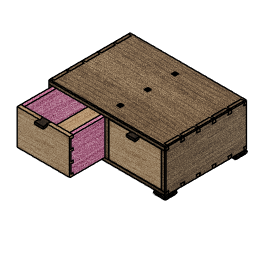
Drawer Box 2019 (Autodesk Fusion 360 design; units mm, degrees)
Autodesk Fusion 360 part; units mm, degrees
note: some values were not read from the file. Chosen so that the rebuilt part matches the saved one: which face or edge a step refers to. Set by a fixed rule: which sketch regions a step uses.
(part 1 of 2)
sketch "Sketch1" plane through (0, 0, 0) normal (0, 1, 0) x (1, 0, 0) in component "Bottom"
  line L0 (0, 0) -> (254, 0)
  line L1 (254, 0) -> (254, -177.8)
  line L2 (254, -177.8) -> (0, -177.8)
  line L3 (0, -177.8) -> (0, 0)
  dimension "d8" = 254
  dimension "d9" = 177.8
  constraint horizontal L0
  constraint vertical L1
  constraint horizontal L2
  constraint vertical L3
  constraint coincident L0.start L3.end
  measures "d8" distance of L1.end L2.end
  measures "d9" distance of L0.start L2.end
extrude "Extrude1" add sketch "Sketch1" along normal blind 15.875 makes body 1 in component "Bottom"
ref_plane "WorkPlane1" through (127, 7.9375, 88.9) normal (1, 0, 0) x (0, 0, -1) in component "Bottom"
ref_plane "WorkPlane3" through (127, 7.9375, 88.9) normal (0, 0, 1) x (1, 0, 0) in component "Bottom"
sketch "Sketch2" plane through (0, 0, 0) normal (-1, 0, 0) x (0, 0, 1) in component "Bottom"
  line L0 (0, 0) -> (177.8, 0)
  line L1 (177.8, 0) -> (177.8, 15.875)
  line L2 (177.8, 15.875) -> (0, 15.875)
  line L3 (0, 15.875) -> (0, 0)
  line L4 (76.2, 15.875) -> (73.6209, 7.9375)
  line L5 (73.6209, 7.9375) -> (104.1791, 7.9375)
  line L6 (104.1791, 7.9375) -> (101.6, 15.875)
  line L7 (144.4625, 15.875) -> (141.8834, 7.9375)
  line L8 (141.8834, 7.9375) -> (172.4416, 7.9375)
  line L9 (172.4416, 7.9375) -> (169.8625, 15.875)
  line L10 (110.3313, 15.875) -> (107.7522, 7.9375)
  line L11 (107.7522, 7.9375) -> (138.3103, 7.9375)
  line L12 (138.3103, 7.9375) -> (135.7312, 15.875)
  line L13 (42.0688, 15.875) -> (39.4897, 7.9375)
  line L14 (39.4897, 7.9375) -> (70.0478, 7.9375)
  line L15 (70.0478, 7.9375) -> (67.4688, 15.875)
  line L16 (7.9375, 15.875) -> (5.3584, 7.9375)
  line L17 (5.3584, 7.9375) -> (35.9166, 7.9375)
  line L18 (35.9166, 7.9375) -> (33.3375, 15.875)
  line L19 (76.2, 15.875) -> (101.6, 15.875)
  line L20 (144.4625, 15.875) -> (169.8625, 15.875)
  line L21 (110.3313, 15.875) -> (135.7312, 15.875)
  line L22 (42.0688, 15.875) -> (67.4688, 15.875)
  line L23 (7.9375, 15.875) -> (33.3375, 15.875)
  dimension "d12" = 72
  dimension "d13" = 72
  dimension "d17" = 68.2625
  dimension "d18" = 0
  dimension "d22" = 25.4
  dimension "d23" = 7.9375
  constraint coincident L2 L4.start
  constraint parallel L2 L5
  constraint coincident L2 L6.end
  constraint parallel L2 L19
  constraint midpoint L2 L19
  measures "d12" angle of L4 L5
  measures "d13" angle of L5 L6
  measures "d22" distance of L4.start L6.end
  measures "d23" distance of L5 L19
extrude "Extrude2" cut sketch "Sketch2" against normal blind 7.9375 contours L2 L16 L17 L18 L23 | L2 L7 L8 L9 L20 | L2 L13 L14 L15 L22 | L2 L10 L11 L12 L21 | L2 L4 L5 L6 L19 bodies 1 in component "Bottom"
mirror "Mirror1" about plane through (127, 7.9375, 88.9) normal (1, 0, 0) of "Extrude2" in component "Bottom"
sketch "Sketch3" plane through (0, 15.875, 0) normal (0, 1, 0) x (-1, 0, 0) in component "Bottom"
  line L0 (-246.0625, 76.2) -> (-254, 76.2)
  line L1 (-254, 76.2) -> (-254, 67.4688)
  line L2 (-254, 67.4688) -> (-246.0625, 67.4688)
  line L3 (-246.0625, 67.4688) -> (-246.0625, 42.0688)
  line L4 (-246.0625, 42.0688) -> (-254, 42.0688)
  line L5 (-254, 42.0688) -> (-254, 33.3375)
  line L6 (-254, 33.3375) -> (-246.0625, 33.3375)
  line L7 (-246.0625, 33.3375) -> (-246.0625, 7.9375)
  line L8 (-246.0625, 7.9375) -> (-254, 7.9375)
  line L9 (-254, 7.9375) -> (-254, 0)
  line L10 (-254, 0) -> (0, 0)
  line L11 (0, 0) -> (0, 7.9375)
  line L12 (0, 7.9375) -> (-7.9375, 7.9375)
  line L13 (-7.9375, 7.9375) -> (-7.9375, 33.3375)
  line L14 (-7.9375, 33.3375) -> (0, 33.3375)
  line L15 (0, 33.3375) -> (0, 42.0688)
  line L16 (0, 42.0688) -> (-7.9375, 42.0688)
  line L17 (-7.9375, 42.0688) -> (-7.9375, 67.4688)
  line L18 (-7.9375, 67.4688) -> (0, 67.4688)
  line L19 (0, 67.4688) -> (0, 76.2)
  line L20 (0, 76.2) -> (-7.9375, 76.2)
  line L21 (-7.9375, 76.2) -> (-7.9375, 101.6)
  line L22 (-7.9375, 101.6) -> (0, 101.6)
  line L23 (0, 101.6) -> (0, 110.3313)
  line L24 (0, 110.3313) -> (-7.9375, 110.3313)
  line L25 (-7.9375, 110.3313) -> (-7.9375, 135.7312)
  line L26 (-7.9375, 135.7313) -> (0, 135.7313)
  line L27 (0, 135.7313) -> (0, 144.4625)
  line L28 (0, 144.4625) -> (-7.9375, 144.4625)
  line L29 (-7.9375, 144.4625) -> (-7.9375, 169.8625)
  line L30 (-7.9375, 169.8625) -> (0, 169.8625)
  line L31 (0, 169.8625) -> (0, 177.8)
  line L32 (0, 177.8) -> (-254, 177.8)
  line L33 (-254, 177.8) -> (-254, 169.8625)
  line L34 (-254, 169.8625) -> (-246.0625, 169.8625)
  line L35 (-246.0625, 169.8625) -> (-246.0625, 144.4625)
  line L36 (-246.0625, 144.4625) -> (-254, 144.4625)
  line L37 (-254, 144.4625) -> (-254, 135.7313)
  line L38 (-254, 135.7313) -> (-246.0625, 135.7313)
  line L39 (-246.0625, 135.7313) -> (-246.0625, 110.3313)
  line L40 (-246.0625, 110.3313) -> (-254, 110.3313)
  line L41 (-254, 110.3313) -> (-254, 101.6)
  line L42 (-254, 101.6) -> (-246.0625, 101.6)
  line L43 (-246.0625, 101.6) -> (-246.0625, 76.2)
  line L44 (-127, 0) -> (-127, 177.8) construction
  line L45 (-123.0312, 84.9313) -> (-130.9688, 84.9313)
  line L46 (-130.9688, 84.9313) -> (-130.9688, 92.8688)
  line L47 (-130.9688, 92.8688) -> (-123.0312, 92.8688)
  line L48 (-123.0312, 92.8688) -> (-123.0312, 84.9313)
  line L49 (-130.9688, 84.9313) -> (-123.0312, 92.8688) construction
  line L50 (-123.0312, 25.6646) -> (-130.9688, 25.6646)
  line L51 (-123.0312, 33.6021) -> (-123.0312, 25.6646)
  line L52 (-130.9688, 33.6021) -> (-123.0312, 33.6021)
  line L53 (-130.9688, 25.6646) -> (-130.9688, 33.6021)
  line L54 (-123.0312, 144.1979) -> (-130.9688, 144.1979)
  line L55 (-123.0312, 152.1354) -> (-123.0312, 144.1979)
  line L56 (-130.9688, 152.1354) -> (-123.0312, 152.1354)
  line L57 (-130.9688, 144.1979) -> (-130.9688, 152.1354)
  dimension "d27" = 7.9375
  dimension "d30" = 59.2667
  dimension "d31" = 0
  constraint midpoint L10 L44.start
  constraint midpoint L32 L44.end
  constraint horizontal L45
  constraint vertical L46
  constraint horizontal L47
  constraint vertical L48
  constraint midpoint L44 L49
  constraint equal L45 L48
  measures "d27" distance of L46.end L47.end
extrude "Extrude3" cut sketch "Sketch3" against normal up to surface (15.875 mm away) contours L45 L46 L47 L48 | L50 L51 L52 L53 | L54 L55 L56 L57 bodies 1 in component "Bottom"
box "BoxPrimitive1" add length 93.6625 width 7.9375 height 177.8 placed x (0, 1, 0) y (-1, 0, 0) z (0, 0, 1) at (7.9375, 0, 0) separate body makes body 2 in component "Side"
ref_plane "WorkPlane1" through (3.9688, 46.8312, 88.9) normal (0, -1, 0) x (0, 0, 1) in component "Side"
sketch "Sketch3 (2)" plane through (0, -32.4835, -5.3174) normal (-1, 0, 0) x (0, 0, 1) in component "Side"
  line L0 (183.1174, 126.146) -> (5.3174, 126.146)
  line L1 (5.3174, 126.146) -> (5.3174, 32.4835)
  line L2 (5.3174, 32.4835) -> (183.1174, 32.4835)
  line L3 (183.1174, 32.4835) -> (183.1174, 126.146)
  line L4 (143.6277, 32.4835) -> (141.0487, 40.421)
  line L5 (47.3862, 40.421) -> (44.8071, 32.4835)
  line L6 (13.2549, 40.421) -> (38.6549, 40.421)
  line L7 (149.7799, 40.421) -> (147.2009, 32.4835)
  line L8 (47.3862, 40.421) -> (72.7862, 40.421)
  line L9 (147.2009, 32.4835) -> (177.759, 32.4835)
  line L10 (13.2549, 40.421) -> (10.6759, 32.4835)
  line L11 (183.1174, 40.421) -> (5.3174, 40.421)
  line L12 (75.3652, 32.4835) -> (72.7862, 40.421)
  line L13 (81.5174, 40.421) -> (106.9174, 40.421)
  line L14 (115.6487, 40.421) -> (113.0696, 32.4835)
  line L15 (109.4965, 32.4835) -> (106.9174, 40.421)
  line L16 (78.9384, 32.4835) -> (109.4965, 32.4835)
  line L17 (41.234, 32.4835) -> (38.6549, 40.421)
  line L18 (10.6759, 32.4835) -> (41.234, 32.4835)
  line L19 (115.6487, 40.421) -> (141.0487, 40.421)
  line L20 (177.759, 32.4835) -> (175.1799, 40.421)
  line L21 (149.7799, 40.421) -> (175.1799, 40.421)
  line L22 (113.0696, 32.4835) -> (143.6277, 32.4835)
  line L23 (44.8071, 32.4835) -> (75.3652, 32.4835)
  line L24 (81.5174, 40.421) -> (78.9384, 32.4835)
  dimension "d42" = 68.2625
  dimension "d43" = 0
  dimension "d44" = 72
  dimension "d45" = 72
  dimension "d46" = 25.4
  dimension "d47" = 7.9375
  constraint coincident L13.start L11
  constraint parallel L11 L16
  constraint coincident L13.end L11
  constraint parallel L11 L13
  constraint midpoint L11 L13
  constraint coincident L1 L11.end
  constraint coincident L2 L10.end
  constraint perpendicular L3 L11
  constraint coincident L3 L11.start
  measures "d44" angle of L16 L24
  measures "d45" angle of L15 L16
  measures "d46" distance of L13.start L13.end
  measures "d47" distance of L13 L16
extrude "Extrude1'" cut sketch "Sketch3 (2)" against normal up to surface (7.9375 mm away) contours L2 L3 L11 L20 | L1 L2 L10 L11 | L2 L4 L7 L11 | L2 L5 L11 L17 | L2 L11 L14 L15 | L2 L11 L12 L24 bodies 2 in component "Side"
mirror "Mirror1'" about plane through (3.9688, 46.8312, 88.9) normal (0, -1, 0) of "Extrude1'" in component "Side"
sketch "Sketch1 (2)" plane through (0, 0, 0) normal (0, 1, 0) x (1, 0, 0) in component "Top"
  line L0 (0, 0) -> (254, 0)
  line L1 (254, 0) -> (254, -177.8)
  line L2 (254, -177.8) -> (0, -177.8)
  line L3 (0, -177.8) -> (0, 0)
  dimension "d8_1" = 254
  dimension "d9_1" = 177.8
  constraint horizontal L0
  constraint vertical L1
  constraint horizontal L2
  constraint vertical L3
  constraint coincident L0.start L3.end
  measures "d8_1" distance of L1.end L2.end
  measures "d9_1" distance of L0.start L2.end
extrude "Extrude1''" add sketch "Sketch1 (2)" along normal blind 7.9375 separate body makes body 3 in component "Top"
ref_plane "WorkPlane1" through (127, 3.9688, 88.9) normal (1, 0, 0) x (0, 0, -1) in component "Top"
sketch "Sketch2 (2)" plane through (0, 0, 0) normal (-1, 0, 0) x (0, 0, 1) in component "Top"
  line L0 (0, 0) -> (177.8, 0)
  line L1 (177.8, 0) -> (177.8, 7.9375)
  line L2 (177.8, 7.9375) -> (0, 7.9375)
  line L3 (0, 7.9375) -> (0, 0)
  line L4 (76.2, 7.9375) -> (73.6209, 0)
  line L5 (73.6209, 0) -> (104.1791, 0)
  line L6 (104.1791, 0) -> (101.6, 7.9375)
  line L7 (144.4625, 7.9375) -> (141.8834, 0)
  line L8 (141.8834, 0) -> (172.4416, 0)
  line L9 (172.4416, 0) -> (169.8625, 7.9375)
  line L10 (110.3313, 7.9375) -> (107.7522, 0)
  line L11 (107.7522, 0) -> (138.3103, 0)
  line L12 (138.3103, 0) -> (135.7313, 7.9375)
  line L13 (42.0688, 7.9375) -> (39.4897, 0)
  line L14 (39.4897, 0) -> (70.0478, 0)
  line L15 (70.0478, 0) -> (67.4688, 7.9375)
  line L16 (7.9375, 7.9375) -> (5.3584, 0)
  line L17 (5.3584, 0) -> (35.9166, 0)
  line L18 (35.9166, 0) -> (33.3375, 7.9375)
  line L19 (76.2, 7.9375) -> (101.6, 7.9375)
  line L20 (144.4625, 7.9375) -> (169.8625, 7.9375)
  line L21 (110.3313, 7.9375) -> (135.7312, 7.9375)
  line L22 (42.0688, 7.9375) -> (67.4688, 7.9375)
  line L23 (7.9375, 7.9375) -> (33.3375, 7.9375)
  dimension "d12_1" = 72
  dimension "d13_1" = 72
  dimension "d17_1" = 68.2625
  dimension "d18_1" = 0
  dimension "d22_1" = 25.4
  dimension "d23_1" = 7.9375
  constraint coincident L2 L4.start
  constraint parallel L2 L5
  constraint coincident L2 L6.end
  constraint parallel L2 L19
  constraint midpoint L2 L19
  measures "d12_1" angle of L4 L5
  measures "d13_1" angle of L5 L6
  measures "d22_1" distance of L4.start L6.end
  measures "d23_1" distance of L5 L19
extrude "Extrude2'" cut sketch "Sketch2 (2)" against normal blind 7.9375 contours L0 L2 L16 L17 L18 L23 | L0 L2 L13 L14 L15 L22 | L0 L2 L4 L5 L6 L19 | L0 L2 L10 L11 L12 L21 | L0 L2 L7 L8 L9 L20 bodies 3 in component "Top"
mirror "Mirror1''" about plane through (127, 3.9688, 88.9) normal (1, 0, 0) of "Extrude2'" in component "Top"
sketch "Sketch3 (3)" plane through (0, 7.9375, 0) normal (0, 1, 0) x (-1, 0, 0) in component "Top"
  line L0 (-246.0625, 76.2) -> (-254, 76.2)
  line L1 (-254, 76.2) -> (-254, 67.4688)
  line L2 (-254, 67.4688) -> (-246.0625, 67.4688)
  line L3 (-246.0625, 67.4688) -> (-246.0625, 42.0688)
  line L4 (-246.0625, 42.0688) -> (-254, 42.0688)
  line L5 (-254, 42.0688) -> (-254, 33.3375)
  line L6 (-254, 33.3375) -> (-246.0625, 33.3375)
  line L7 (-246.0625, 33.3375) -> (-246.0625, 7.9375)
  line L8 (-246.0625, 7.9375) -> (-254, 7.9375)
  line L9 (-254, 7.9375) -> (-254, 0)
  line L10 (-254, 0) -> (0, 0)
  line L11 (0, 0) -> (0, 7.9375)
  line L12 (0, 7.9375) -> (-7.9375, 7.9375)
  line L13 (-7.9375, 7.9375) -> (-7.9375, 33.3375)
  line L14 (-7.9375, 33.3375) -> (0, 33.3375)
  line L15 (0, 33.3375) -> (0, 42.0688)
  line L16 (0, 42.0688) -> (-7.9375, 42.0688)
  line L17 (-7.9375, 42.0688) -> (-7.9375, 67.4688)
  line L18 (-7.9375, 67.4688) -> (0, 67.4688)
  line L19 (0, 67.4688) -> (0, 76.2)
  line L20 (0, 76.2) -> (-7.9375, 76.2)
  line L21 (-7.9375, 76.2) -> (-7.9375, 101.6)
  line L22 (-7.9375, 101.6) -> (0, 101.6)
  line L23 (0, 101.6) -> (0, 110.3313)
  line L24 (0, 110.3313) -> (-7.9375, 110.3313)
  line L25 (-7.9375, 110.3313) -> (-7.9375, 135.7312)
  line L26 (-7.9375, 135.7313) -> (0, 135.7313)
  line L27 (0, 135.7313) -> (0, 144.4625)
  line L28 (0, 144.4625) -> (-7.9375, 144.4625)
  line L29 (-7.9375, 144.4625) -> (-7.9375, 169.8625)
  line L30 (-7.9375, 169.8625) -> (0, 169.8625)
  line L31 (0, 169.8625) -> (0, 177.8)
  line L32 (0, 177.8) -> (-254, 177.8)
  line L33 (-254, 177.8) -> (-254, 169.8625)
  line L34 (-254, 169.8625) -> (-246.0625, 169.8625)
  line L35 (-246.0625, 169.8625) -> (-246.0625, 144.4625)
  line L36 (-246.0625, 144.4625) -> (-254, 144.4625)
  line L37 (-254, 144.4625) -> (-254, 135.7313)
  line L38 (-254, 135.7313) -> (-246.0625, 135.7313)
  line L39 (-246.0625, 135.7313) -> (-246.0625, 110.3313)
  line L40 (-246.0625, 110.3313) -> (-254, 110.3313)
  line L41 (-254, 110.3313) -> (-254, 101.6)
  line L42 (-254, 101.6) -> (-246.0625, 101.6)
  line L43 (-246.0625, 101.6) -> (-246.0625, 76.2)
  line L44 (-127, 0) -> (-127, 177.8) construction
  line L45 (-123.0312, 84.9313) -> (-130.9688, 84.9313)
  line L46 (-130.9688, 84.9313) -> (-130.9688, 92.8688)
  line L47 (-130.9688, 92.8688) -> (-123.0312, 92.8688)
  line L48 (-123.0312, 92.8688) -> (-123.0312, 84.9313)
  line L49 (-130.9688, 84.9313) -> (-123.0312, 92.8688) construction
  line L50 (-123.0312, 25.6646) -> (-130.9688, 25.6646)
  line L51 (-123.0312, 33.6021) -> (-123.0312, 25.6646)
  line L52 (-130.9688, 33.6021) -> (-123.0312, 33.6021)
  line L53 (-130.9688, 25.6646) -> (-130.9688, 33.6021)
  line L54 (-123.0312, 144.1979) -> (-130.9688, 144.1979)
  line L55 (-123.0312, 152.1354) -> (-123.0312, 144.1979)
  line L56 (-130.9688, 152.1354) -> (-123.0312, 152.1354)
  line L57 (-130.9688, 144.1979) -> (-130.9688, 152.1354)
  dimension "d27_1" = 7.9375
  dimension "d30_1" = 59.2667
  dimension "d31_1" = 0
  constraint midpoint L10 L44.start
  constraint midpoint L32 L44.end
  constraint horizontal L45
  constraint vertical L46
  constraint horizontal L47
  constraint vertical L48
  constraint midpoint L44 L49
  constraint equal L45 L48
  measures "d27_1" distance of L46.end L47.end
extrude "Extrude3'" cut sketch "Sketch3 (3)" against normal up to surface (7.9375 mm away) contours L45 L46 L47 L48 | L50 L51 L52 L53 | L54 L55 L56 L57 bodies 3 in component "Top"
sketch "Sketch1 (3)" plane through (0, 0, 0) normal (1, 0, 0) x (0, 0, -1) in component "Divider"
  line L0 (-169.8625, 0) -> (-169.8625, 77.7875)
  line L1 (0, 77.7875) -> (0, 0)
  line L2 (-76.9938, 77.7875) -> (-76.9938, 85.725)
  line L3 (-76.9938, 85.725) -> (-84.9313, 85.725)
  line L4 (-84.9313, 85.725) -> (-84.9313, 77.7875)
  line L5 (-80.9625, 85.725) -> (-80.9625, -7.9375) construction
  line L6 (-169.8625, 38.8937) -> (0, 38.8937) construction
  line L7 (-136.2604, 77.7875) -> (-136.2604, 85.725)
  line L8 (-144.1979, 85.725) -> (-144.1979, 77.7875)
  line L9 (-136.2604, 85.725) -> (-144.1979, 85.725)
  line L10 (-17.7271, 77.7875) -> (-17.7271, 85.725)
  line L11 (-25.6646, 85.725) -> (-25.6646, 77.7875)
  line L12 (-17.7271, 85.725) -> (-25.6646, 85.725)
  line L13 (-76.9938, 77.7875) -> (-25.6646, 77.7875)
  line L14 (-17.7271, 77.7875) -> (0, 77.7875)
  line L15 (-169.8625, 77.7875) -> (-144.1979, 77.7875)
  line L16 (-136.2604, 77.7875) -> (-84.9313, 77.7875)
  line L17 (0, 0) -> (-17.7271, 0)
  line L18 (-76.9937, 0) -> (-76.9938, -7.9375)
  line L19 (-76.9938, -7.9375) -> (-84.9313, -7.9375)
  line L20 (-84.9313, -7.9375) -> (-84.9313, 0)
  line L21 (-136.2604, -7.9375) -> (-144.1979, -7.9375)
  line L22 (-136.2604, 0) -> (-136.2604, -7.9375)
  line L23 (-144.1979, -7.9375) -> (-144.1979, 0)
  line L24 (-17.7271, -7.9375) -> (-25.6646, -7.9375)
  line L25 (-17.7271, 0) -> (-17.7271, -7.9375)
  line L26 (-25.6646, -7.9375) -> (-25.6646, 0)
  line L27 (-76.9937, 0) -> (-25.6646, 0)
  line L28 (-17.7271, 0) -> (0, 0)
  line L29 (-169.8625, 0) -> (-144.1979, 0)
  line L30 (-136.2604, 0) -> (-84.9313, 0)
  point P0 (-140.2292, 85.725)
  point P1 (-21.6958, 85.725)
  point P2 (-140.2292, -7.9375)
  point P3 (-21.6958, -7.9375)
  dimension "d87" = 169.8625
  dimension "d88" = 77.7875
  dimension "d89" = 7.9375
  dimension "d90" = 88.9
  dimension "d91" = 80.9625
  dimension "d94" = 59.2667
  dimension "d95" = 0
  dimension "d99" = 7.9375
  dimension "d102" = 59.2667
  dimension "d103" = 0
  constraint horizontal L17
  constraint vertical L0
  constraint horizontal L15
  constraint vertical L1
  constraint coincident L1.end L17.start
  constraint vertical L2
  constraint horizontal L3
  constraint vertical L4
  constraint collinear L13 L15
  constraint equal L3 L4
  constraint midpoint L3 L5.start
  constraint midpoint L0 L6.start
  constraint midpoint L1 L6.end
  constraint collinear L13 L14
  constraint collinear L15 L16
  constraint perpendicular L1 L29
  constraint vertical L18
  constraint horizontal L19
  constraint vertical L20
  constraint collinear L27 L29
  constraint midpoint L5.end L19
  constraint collinear L4 L20
  constraint collinear L27 L28
  constraint collinear L29 L30
  measures "d87" distance of L1.end L0.start
  measures "d88" distance of L1.end L1.start
  measures "d89" distance of L4.end L3.end
  measures "d90" distance of L0 L5
  measures "d91" distance of L1 L5
  measures "d99" distance of L20.end L19.end
extrude "Extrude1'''" add sketch "Sketch1 (3)" along normal blind 7.9375 separate body makes body 4 in component "Divider"
sketch "Sketch2 (3)" plane through (0, 0, 144.1979) normal (0, 0, 1) x (1, 0, 0) in component "Divider"
  line L0 (0, 85.725) -> (0, 77.7875)
  line L1 (0, 77.7875) -> (7.9375, 77.7875)
  line L2 (7.9375, 77.7875) -> (7.9375, 85.725)
  line L3 (7.9375, 85.725) -> (0, 85.725)
  line L4 (1.1906, 85.725) -> (2.7781, 85.725)
  line L5 (2.7781, 85.725) -> (2.7781, 79.375)
  line L6 (2.7781, 79.375) -> (1.1906, 79.375)
  line L7 (1.1906, 79.375) -> (1.1906, 85.725)
  line L8 (0, -7.9375) -> (7.9375, -7.9375)
  line L9 (3.9688, -7.9375) -> (3.9688, 85.725) construction
  line L10 (2.7781, 85.725) -> (3.9688, 85.725) construction
  line L11 (1.1906, 85.725) -> (0, 85.725) construction
  line L12 (1.1906, -7.9375) -> (2.7781, -7.9375)
  line L13 (2.7781, -7.9375) -> (2.7781, -1.5875)
  line L14 (2.7781, -1.5875) -> (1.1906, -1.5875)
  line L15 (1.1906, -1.5875) -> (1.1906, -7.9375)
  line L16 (6.7469, 85.725) -> (5.1594, 85.725)
  line L17 (5.1594, 79.375) -> (6.7469, 79.375)
  line L18 (5.1594, 85.725) -> (5.1594, 79.375)
  line L19 (6.7469, 79.375) -> (6.7469, 85.725)
  line L20 (5.1594, -7.9375) -> (5.1594, -1.5875)
  line L21 (6.7469, -1.5875) -> (6.7469, -7.9375)
  line L22 (5.1594, -1.5875) -> (6.7469, -1.5875)
  line L23 (6.7469, -7.9375) -> (5.1594, -7.9375)
  dimension "d105" = 1.5875
  dimension "d106" = 6.35
  dimension "d107" = 1.5875
  dimension "d108" = 6.35
  constraint horizontal L4
  constraint vertical L5
  constraint horizontal L6
  constraint vertical L7
  constraint coincident L3 L4.start
  constraint midpoint L8 L9.start
  constraint midpoint L3 L9.end
  constraint coincident L0.start L3.end
  constraint equal L10 L11
  constraint horizontal L12
  constraint vertical L13
  constraint horizontal L14
  constraint vertical L15
  constraint coincident L8 L12.start
  constraint collinear L7 L15
  constraint symmetric L4.start L9 L16.start
  constraint symmetric L4.end L9 L16.end
  constraint symmetric L5.end L9 L17.start
  constraint symmetric L6.end L9 L17.end
  constraint symmetric L9 L12.start L21.end
  constraint symmetric L9 L12.end L20.start
  constraint symmetric L9 L13.end L20.end
  constraint symmetric L9 L14.end L21.start
  measures "d105" distance of L4.start L4.end
  measures "d106" distance of L4.start L6.end
  measures "d107" distance of L12.start L12.end
  measures "d108" distance of L12.start L14.end
extrude "Extrude2''" cut sketch "Sketch2 (3)" against normal up to surface (126.4708 mm away) contours L3 L4 L5 L6 L7 | L3 L16 L17 L18 L19 | L8 L12 L13 L14 L15 | L8 L20 L21 L22 L23 bodies 4 in component "Divider"
sketch "Sketch4" plane through (0, 0, 0) normal (0, 0, -1) x (-1, 0, 0) in component "Side"
  line L0 (0, 85.725) -> (-7.9375, 85.725)
  line L1 (-7.9375, 85.725) -> (-7.9375, 7.9375)
  line L2 (-7.9375, 7.9375) -> (0, 7.9375)
  line L3 (0, 7.9375) -> (0, 85.725)
  line L4 (-3.9688, 85.725) -> (0, 85.725)
  line L5 (0, 85.725) -> (0, 7.9375)
  line L6 (0, 7.9375) -> (-3.9688, 7.9375)
  line L7 (-3.9688, 7.9375) -> (-3.9688, 85.725)
  constraint horizontal L4
  constraint vertical L5
  constraint horizontal L6
  constraint vertical L7
  constraint coincident L2.end L3.start
  constraint midpoint L0 L4.start
extrude "Extrude2'''" cut sketch "Sketch4" against normal blind 7.9375 contours L0 L2 L3 L4 L5 L6 L7 bodies 2 in component "Side"
sketch "Sketch1 (4)" plane through (0, 0, 0) normal (0, 0, 1) x (1, 0, 0) in component "Back"
  line L0 (0, 0) -> (246.0625, 0)
  line L1 (246.0625, 0) -> (246.0625, 77.7875)
  line L2 (246.0625, 77.7875) -> (0, 77.7875)
  line L3 (0, 77.7875) -> (0, 0)
  dimension "d149" = 246.0625
  dimension "d150" = 77.7875
  constraint horizontal L0
  constraint vertical L1
  constraint horizontal L2
  constraint vertical L3
  constraint coincident L0.start L3.end
  measures "d149" distance of L0.start L0.end
  measures "d150" distance of L0.start L2.end
extrude "Extrude1''''" add sketch "Sketch1 (4)" along normal blind 7.9375 separate body makes body 5 in component "Back"
sketch "Sketch4 (2)" plane through (0, 0, 0) normal (0, -1, 0) x (1, 0, 0) in component "Bottom"
  line L0 (130.9688, 33.6021) -> (130.9688, 25.6646)
  line L1 (130.9688, 25.6646) -> (123.0312, 25.6646)
  line L2 (123.0312, 25.6646) -> (123.0312, 33.6021)
  line L3 (123.0312, 33.6021) -> (130.9688, 33.6021)
  line L4 (123.0312, 84.9313) -> (123.0312, 92.8688)
  line L5 (123.0312, 92.8688) -> (130.9688, 92.8688)
  line L6 (130.9688, 92.8688) -> (130.9688, 84.9313)
  line L7 (130.9688, 84.9313) -> (123.0312, 84.9313)
  line L8 (130.9688, 152.1354) -> (130.9688, 144.1979)
  line L9 (130.9688, 144.1979) -> (123.0312, 144.1979)
  line L10 (123.0312, 144.1979) -> (123.0312, 152.1354)
  line L11 (123.0312, 152.1354) -> (130.9688, 152.1354)
  line L12 (254, 177.8) -> (0, 177.8)
  line L13 (0, 177.8) -> (0, 0)
  line L14 (0, 0) -> (254, 0)
  line L15 (254, 0) -> (254, 177.8)
  line L16 (0, 177.8) -> (25.4, 177.8)
  line L17 (25.4, 177.8) -> (25.4, 152.4)
  line L18 (25.4, 152.4) -> (0, 152.4)
  line L19 (0, 152.4) -> (0, 177.8)
  line L20 (127, 177.8) -> (127, 0) construction
  line L21 (0, 88.9) -> (254, 88.9) construction
  line L22 (254, 177.8) -> (228.6, 177.8)
  line L23 (254, 152.4) -> (254, 177.8)
  line L24 (228.6, 177.8) -> (228.6, 152.4)
  line L25 (228.6, 152.4) -> (254, 152.4)
  line L26 (0, 25.4) -> (0, 0)
  line L27 (25.4, 0) -> (25.4, 25.4)
  line L28 (25.4, 25.4) -> (0, 25.4)
  line L29 (0, 0) -> (25.4, 0)
  line L30 (228.6, 25.4) -> (254, 25.4)
  line L31 (254, 25.4) -> (254, 0)
  line L32 (228.6, 0) -> (228.6, 25.4)
  line L33 (254, 0) -> (228.6, 0)
  point P0 (254, 177.8)
  point P1 (254, 0)
  point P2 (254, 0)
  dimension "d166" = 25.4
  constraint horizontal L16
  constraint vertical L17
  constraint horizontal L18
  constraint vertical L19
  constraint coincident L12.end L13.start
  constraint midpoint L12 L20.start
  constraint midpoint L14 L20.end
  constraint midpoint L13 L21.start
  constraint midpoint L15 L21.end
  constraint equal L16 L19
  constraint symmetric L12.end L20 P0
  constraint symmetric L16.end L20 L22.end
  constraint symmetric L17.end L20 L24.end
  constraint symmetric L18.end L20 L23.start
  constraint symmetric P0 L21 P2
  constraint symmetric L12.end L21 L13.end
  constraint symmetric L16.end L21 L27.start
  constraint symmetric L17.end L21 L27.end
  constraint symmetric L18.end L21 L26.start
  constraint symmetric L21 L22.end L32.start
  constraint symmetric L21 L23.start L30.end
  constraint symmetric L21 P0 P2
  constraint symmetric L21 L24.end L30.start
  measures "d166" distance of L12.end L16.end
extrude "Extrude4" cut sketch "Sketch4 (2)" against normal blind 7.9375 contours L12 L13 L14 L15 L17 L18 L24 L25 L27 L28 L30 L32 bodies 1 in component "Bottom"
sketch "Sketch5" plane through (0, 0, 0) normal (-1, 0, 0) x (0, 0, 1) in component "Bottom"
  line L0 (152.4, 7.9375) -> (152.4, 0)
  line L1 (152.4, 0) -> (177.8, 0)
  line L2 (177.8, 0) -> (177.8, 15.875)
  line L3 (177.8, 15.875) -> (169.8625, 15.875)
  line L4 (169.8625, 15.875) -> (172.4416, 7.9375)
  line L5 (172.4416, 7.9375) -> (152.4, 7.9375)
  line L6 (176.2125, 7.9375) -> (177.8, 7.9375)
  arc A0 (176.2125, 0.7937) -> (176.2125, 7.1438) centre (173.8313, 3.9688) ccw
  line L7 (176.2125, 7.9375) -> (176.2125, 7.1438)
  line L8 (176.2125, 0) -> (176.2125, 0.7937)
  line L9 (176.2125, 7.1437) -> (177.8, 5.5562)
  line L10 (176.2125, 0.7937) -> (177.8, 2.3813)
  dimension "d171" = 3.9688
  dimension "d172" = 0.7937
  dimension "d451" = 135
  dimension "d452" = 135
  dimension "d453" = 1.5875
  constraint tangent L2 A0
  constraint tangent L1 A0
  constraint midpoint L2 L6.end
  constraint tangent L6 A0
  constraint perpendicular L6 L7
  constraint coincident L1 L8.start
  constraint perpendicular L1 L8
  constraint collinear L7 L8
  constraint coincident L2 L9.end
  constraint coincident L2 L10.end
  measures "d171" radius of A0
  measures "d172" distance of L6.start L9.start
  measures "d451" angle of L7 L9
  measures "d452" angle of L8 L10
  measures "d453" distance of L1.end L8.start
sweep "Sweep1" cut profiles "Sketch5" along 4 edges at (25.4, 0, 165.1) (12.7, 0, 177.8) (0, 0, 165.1) (12.7, 0, 152.4) section 1 contours L1 L2 A0 L8 L10 | A0 L10 | L2 L6 A0 L7 L9 | A0 L9 on bodies 1 bodies 1 in component "Bottom"
mirror "Mirror3" about plane through (127, 7.9375, 88.9) normal (1, 0, 0) of "Sweep1" in component "Bottom"
mirror "Mirror4" about plane through (127, 7.9375, 88.9) normal (0, 0, 1) of "Sweep1", "Mirror3" in component "Bottom"
sketch "Sketch1 (5)" plane through (0, 0, 0) normal (0, 0, 1) x (1, 0, 0) in component "DrawerFront"
  line L0 (0, 0) -> (113.5062, 0)
  line L1 (113.5062, 0) -> (113.5062, 76.9938)
  line L2 (113.5062, 76.9938) -> (0, 76.9938)
  line L3 (0, 76.9938) -> (0, 0)
  dimension "d187" = 76.9938
  dimension "d188" = 113.5062
  constraint horizontal L0
  constraint vertical L1
  constraint horizontal L2
  constraint vertical L3
  constraint coincident L0.start L3.end
  measures "d187" distance of L0.start L2.end
  measures "d188" distance of L0.start L0.end
extrude "Extrude1'''''" add sketch "Sketch1 (5)" along normal blind 7.9375 separate body makes body 6 in component "DrawerFront"
ref_plane "WorkPlane1" through (56.7531, 38.4969, 3.9688) normal (1, 0, 0) x (0, 1, 0) in component "DrawerFront"
sketch "Sketch2 (4)" plane through (0, 0, 0) normal (-1, 0, 0) x (0, 0, 1) in component "DrawerFront"
  line L0 (0, 76.9938) -> (0, 0)
  line L1 (0, 0) -> (7.9375, 0)
  line L2 (7.9375, 0) -> (7.9375, 76.9938)
  line L3 (7.9375, 76.9938) -> (0, 76.9938)
  line L4 (0, 47.2281) -> (4.7625, 48.7756)
  line L5 (4.7625, 48.7756) -> (4.7625, 28.2182)
  line L6 (4.7625, 28.2182) -> (0, 29.7656)
  line L7 (0, 29.7656) -> (0, 47.2281)
  line L8 (0, 53.1813) -> (0, 70.6438)
  line L9 (0, 70.6437) -> (4.7625, 72.1912)
  line L10 (4.7625, 72.1912) -> (4.7625, 51.6338)
  line L11 (4.7625, 51.6338) -> (0, 53.1813)
  line L12 (0, 6.35) -> (0, 23.8125)
  line L13 (0, 23.8125) -> (4.7625, 25.3599)
  line L14 (4.7625, 25.3599) -> (4.7625, 4.8026)
  line L15 (4.7625, 4.8026) -> (0, 6.35)
  dimension "d191" = 4.7625
  dimension "d192" = 108
  dimension "d193" = 108
  dimension "d197" = 17.4625
  dimension "d202" = 23.4156
  dimension "d203" = 0
  constraint coincident L0 L4.start
  constraint parallel L0 L5
  constraint coincident L0 L6.end
  constraint midpoint L0 L7
  measures "d191" distance of L5 L7
  measures "d192" angle of L4 L7
  measures "d193" angle of L6 L7
  measures "d197" distance of L4.start L6.end
extrude "Extrude2''''" cut sketch "Sketch2 (4)" against normal blind 7.9375 contours L0 L8 L9 L10 L11 | L0 L4 L5 L6 L7 | L0 L12 L13 L14 L15 bodies 6 in component "DrawerFront"
mirror "Mirror1'''" about plane through (56.7531, 38.4969, 3.9688) normal (1, 0, 0) of "Extrude2''''" in component "DrawerFront"
sketch "Sketch3 (4)" plane through (0, 76.9938, 0) normal (0, 1, 0) x (-1, 0, 0) in component "DrawerFront"
  line L0 (-113.5062, 0) -> (0, 0)
  line L1 (0, 0) -> (0, 7.9375)
  line L2 (0, 7.9375) -> (-113.5062, 7.9375)
  line L3 (-113.5062, 7.9375) -> (-113.5062, 0)
  line L4 (-49.8072, 7.9375) -> (-47.2281, 0)
  line L5 (-63.6991, 7.9375) -> (-66.2781, 0)
  line L6 (-49.8072, 7.9375) -> (-63.6991, 7.9375)
  dimension "d208" = 19.05
  dimension "d209" = 108
  dimension "d210" = 108
  constraint coincident L2 L4.start
  constraint coincident L0 L4.end
  constraint coincident L2 L5.start
  constraint coincident L0 L5.end
  constraint midpoint L2 L6
  measures "d208" distance of L4.end L5.end
  measures "d209" angle of L2 L4
  measures "d210" angle of L2 L5
extrude "Extrude3''" cut sketch "Sketch3 (4)" against normal blind 4.7625 contours L0 L2 L4 L5 L6 bodies 6 in component "DrawerFront"
chamfer "Chamfer1" distance 0.7937 angle 45 1 edges at (56.7531, 0, 7.9375) on bodies 6 in component "DrawerFront"
sketch "Sketch1 (6)" plane through (0, 0, 0) normal (1, 0, 0) x (0, 0, -1) in component "DrawerSide"
  line L0 (0, 0) -> (166.6875, 0)
  line L1 (166.6875, 0) -> (166.6875, 76.9938)
  line L2 (166.6875, 76.9938) -> (0, 76.9938)
  line L3 (0, 76.9938) -> (0, 0)
  dimension "d216" = 76.9938
  dimension "d217" = 166.6875
  constraint horizontal L0
  constraint vertical L1
  constraint horizontal L2
  constraint vertical L3
  constraint coincident L0.start L3.end
  measures "d216" distance of L0.end L1.end
  measures "d217" distance of L1.end L2.end
extrude "Extrude1''''''" add sketch "Sketch1 (6)" along normal blind 7.9375 separate body makes body 7 in component "DrawerSide"
sketch "Sketch3 (5)" plane through (0, 0, 0) normal (-1, 0, 0) x (0, 0, 1) in component "DrawerSide"
  line L0 (0, 0) -> (0, 76.9938)
  line L1 (0, 76.9938) -> (-166.6875, 76.9938)
  line L2 (-166.6875, 76.9938) -> (-166.6875, 0)
  line L3 (-166.6875, 0) -> (0, 0)
  line L4 (0, 28.2182) -> (-4.7625, 29.7656)
  line L5 (-4.7625, 70.6438) -> (0, 72.1912)
  line L6 (-4.7625, 6.35) -> (-4.7625, 23.8125)
  line L7 (0, 4.8026) -> (-4.7625, 6.35)
  line L8 (0, 72.1912) -> (0, 51.6338)
  line L9 (-4.7625, 29.7656) -> (-4.7625, 47.2281)
  line L10 (0, 51.6338) -> (-4.7625, 53.1813)
  line L11 (-4.7625, 23.8125) -> (0, 25.3599)
  line L12 (-4.7625, 53.1813) -> (-4.7625, 70.6438)
  line L13 (0, 48.7756) -> (0, 28.2182)
  line L14 (0, 25.3599) -> (0, 4.8026)
  line L15 (-4.7625, 47.2281) -> (0, 48.7756)
  line L16 (-4.7625, 70.6438) -> (-4.7625, 76.9938)
  line L17 (-4.7625, 53.1813) -> (-4.7625, 47.2281)
  line L18 (-4.7625, 29.7656) -> (-4.7625, 23.8125)
  line L19 (-4.7625, 6.35) -> (-4.7625, 0)
  line L20 (-158.75, 69.0562) -> (-158.75, 31.3531)
  line L21 (-158.75, 7.9375) -> (-166.6875, 5.3584)
  line L22 (-166.6875, 24.8041) -> (-158.75, 22.225)
  line L23 (-158.75, 22.225) -> (-158.75, 76.9938)
  line L24 (-166.6875, 71.6353) -> (-158.75, 69.0562)
  line L25 (-166.6875, 5.3584) -> (-166.6875, 24.8041)
  line L26 (-158.75, 69.0562) -> (-158.75, 54.7687)
  line L27 (-158.75, 45.6406) -> (-158.75, 31.3531)
  line L28 (-166.6875, 76.9938) -> (-166.6875, 0)
  line L29 (-158.75, 54.7687) -> (-158.75, 0)
  line L30 (-158.75, 54.7687) -> (-166.6875, 52.1897)
  line L31 (-166.6875, 52.1897) -> (-166.6875, 71.6353)
  line L32 (-158.75, 22.225) -> (-158.75, 7.9375)
  line L33 (-158.75, 31.3531) -> (-166.6875, 28.7741)
  line L34 (-166.6875, 48.2197) -> (-158.75, 45.6406)
  line L35 (-166.6875, 28.7741) -> (-166.6875, 48.2197)
  line L36 (-158.75, 45.6406) -> (-158.75, 7.9375)
  point P0 (97.155, 99.2187)
  dimension "d222" = 23.4156
  dimension "d223" = 0
  dimension "d224" = 4.7625
  dimension "d225" = 108
  dimension "d226" = 108
  dimension "d227" = 17.4625
  dimension "d230" = 23.4156
  dimension "d231" = 0
  dimension "d232" = 7.9375
  dimension "d233" = 108
  dimension "d234" = 108
  dimension "d235" = 14.2875
  constraint coincident L0 L5.end
  constraint midpoint L0 L13
  constraint coincident L1 L16.end
  constraint perpendicular L1 L16
  constraint coincident L3 L19.end
  constraint perpendicular L3 L19
  constraint coincident L30.end L28
  constraint midpoint L28 L35
  constraint coincident L2.end L3.start
  constraint coincident L2 L1.end
  constraint coincident L1.end L2.start
  constraint vertical L23
  constraint coincident L1 L23.end
  constraint vertical L29
  constraint coincident L3 L29.end
  measures "d224" distance of L9 L13
  measures "d225" angle of L9 L15
  measures "d226" angle of L4 L9
  measures "d227" distance of L9.end L4.end
  measures "d232" distance of L27 L35
  measures "d233" angle of L27 L33
  measures "d234" angle of L27 L34
  measures "d235" distance of L20.end L27.start
extrude "Extrude2'''''" cut sketch "Sketch3 (5)" against normal up to surface (7.9375 mm away) contours L0 L3 L7 L19 | L0 L4 L11 L18 | L0 L10 L15 L17 | L2 L22 L23 L28 L29 L33 L36 | L0 L1 L5 L16 | L2 L20 L23 L28 L29 L30 L34 | L1 L2 L23 L24 L28 bodies 7 in component "DrawerSide"
sketch "Sketch5 (2)" plane through (0, 0, 0) normal (0, -1, 0) x (1, 0, 0) in component "DrawerSide"
  line L0 (7.9375, -4.7625) -> (0, -4.7625)
  line L1 (0, -4.7625) -> (0, -166.6875)
  line L2 (0, -166.6875) -> (7.9375, -166.6875)
  line L3 (7.9375, -166.6875) -> (7.9375, -4.7625)
  line L4 (7.9375, -4.7625) -> (3.9688, -4.7625)
  line L5 (3.9688, -4.7625) -> (3.9688, -166.6875)
  line L6 (3.9688, -166.6875) -> (7.9375, -166.6875)
  line L7 (7.9375, -166.6875) -> (7.9375, -4.7625)
  constraint horizontal L4
  constraint vertical L5
  constraint horizontal L6
  constraint vertical L7
  constraint midpoint L2 L5.end
  constraint coincident L0.start L3.end
extrude "Extrude4'" cut sketch "Sketch5 (2)" against normal blind 7.9375 contours L0 L2 L3 L4 L5 L6 L7 bodies 7 in component "DrawerSide"
sketch "Sketch1 (7)" plane through (0, 0, 0) normal (0, 0, 1) x (1, 0, 0) in component "DrawerBack"
  line L0 (0, 0) -> (113.5062, 0)
  line L1 (113.5062, 0) -> (113.5062, 69.0563)
  line L2 (113.5062, 69.0563) -> (0, 69.0563)
  line L3 (0, 69.0563) -> (0, 0)
  dimension "d242" = 113.5062
  dimension "d243" = 69.0563
  constraint horizontal L0
  constraint vertical L1
  constraint horizontal L2
  constraint vertical L3
  constraint coincident L0.start L3.end
  measures "d242" distance of L0.start L0.end
  measures "d243" distance of L0.start L2.end
extrude "Extrude1'''''''" add sketch "Sketch1 (7)" along normal blind 7.9375 separate body makes body 8 in component "DrawerBack"
ref_plane "WorkPlane1" through (56.7531, 34.5281, 3.9688) normal (-1, 0, 0) x (0, -1, 0) in component "DrawerBack"
sketch "Sketch2 (5)" plane through (0, 0, 0) normal (-1, 0, 0) x (0, 0, 1) in component "DrawerBack"
  line L0 (0, 69.0563) -> (0, 0)
  line L1 (0, 0) -> (7.9375, 0)
  line L2 (7.9375, 0) -> (7.9375, 69.0563)
  line L3 (7.9375, 69.0563) -> (0, 69.0563)
  line L4 (0, 16.8666) -> (7.9375, 14.2875)
  line L5 (7.9375, 46.8312) -> (0, 44.2522)
  line L6 (0, 69.0563) -> (0, -2.5791)
  line L7 (0, 63.6978) -> (7.9375, 61.1188)
  line L8 (7.9375, 23.4156) -> (0, 20.8366)
  line L9 (7.9375, 61.1188) -> (7.9375, 46.8312)
  line L10 (7.9375, 0) -> (0, -2.5791)
  line L11 (0, -2.5791) -> (0, 16.8666)
  line L12 (7.9375, 61.1188) -> (7.9375, 23.4156)
  line L13 (0, 20.8366) -> (0, 40.2822)
  line L14 (7.9375, 46.8312) -> (7.9375, 0)
  line L15 (0, 69.0563) -> (0, -2.5791)
  line L16 (0, 40.2822) -> (7.9375, 37.7031)
  line L17 (7.9375, 37.7031) -> (7.9375, 23.4156)
  line L18 (7.9375, 14.2875) -> (7.9375, 69.0563)
  line L19 (7.9375, 14.2875) -> (7.9375, 0)
  line L20 (0, 44.2522) -> (0, 63.6978)
  line L21 (7.9375, 37.7031) -> (7.9375, 0)
  dimension "d248" = 23.4156
  dimension "d249" = 0
  dimension "d250" = 7.9375
  dimension "d251" = 108
  dimension "d252" = 108
  dimension "d253" = 14.2875
  dimension "d255" = 7.9375
  constraint coincident L5.end L15
  constraint coincident L0.start L6
  constraint coincident L0.start L3.end
  constraint vertical L18
  constraint vertical L14
  constraint coincident L2 L3.start
  constraint coincident L2.end L3.start
  measures "d250" distance of L13 L17
  measures "d251" angle of L8 L17
  measures "d252" angle of L16 L17
  measures "d253" distance of L8.start L16.end
  measures "d255" distance of L7.end L2.end
extrude "Extrude2''''''" cut sketch "Sketch2 (5)" against normal blind 7.9375 contours L0 L2 L5 L6 L7 L9 L12 L15 L18 L20 | L0 L2 L6 L8 L12 L13 L14 L15 L16 L17 L18 L21 | L0 L1 L2 L4 L6 L11 L14 L15 L19 L21 bodies 8 in component "DrawerBack"
mirror "Mirror1''''" about plane through (56.7531, 34.5281, 3.9688) normal (-1, 0, 0) of "Extrude2''''''" in component "DrawerBack"
mirror "MirrorComponent1" about plane through (0, 0, 0) normal (0, 0, 1) of bodies 7 makes body 9 in component "DrawerSide(Mirror)"
sketch "Sketch1 (8)" plane through (0, 0, 0) normal (0, 1, 0) x (1, 0, 0) in component "DrawerBottom"
  line L0 (0, 0) -> (105.5687, 0)
  line L1 (105.5687, 0) -> (105.5687, 161.925)
  line L2 (105.5687, 161.925) -> (0, 161.925)
  line L3 (0, 161.925) -> (0, 0)
  dimension "d295" = 105.5688
  dimension "d296" = 161.925
  constraint horizontal L0
  constraint vertical L1
  constraint horizontal L2
  constraint vertical L3
  constraint coincident L0.start L3.end
  measures "d295" distance of L0.start L0.end
  measures "d296" distance of L0.end L1.end
extrude "Extrude1''''''''" add sketch "Sketch1 (8)" along normal blind 7.9375 separate body makes body 10 in component "DrawerBottom"
sketch "Sketch1 (9)" plane through (0, 0, 0) normal (0, 1, 0) x (1, 0, 0) in component "Pull"
  line L0 (0, 0) -> (19.05, 0)
  line L1 (19.05, -7.9375) -> (19.05, -17.4625)
  line L2 (19.05, -17.4625) -> (0, -17.4625)
  line L3 (0, -17.4625) -> (0, -7.9375)
  line L4 (0, 0) -> (2.5791, -7.9375)
  line L5 (2.5791, -7.9375) -> (0, -7.9375)
  line L6 (19.05, 0) -> (16.4709, -7.9375)
  line L7 (16.4709, -7.9375) -> (19.05, -7.9375)
  dimension "d340" = 19.05
  dimension "d341" = 17.4625
  dimension "d342" = 72
  dimension "d343" = 72
  dimension "d344" = 7.9375
  constraint horizontal L0
  constraint vertical L1
  constraint horizontal L2
  constraint vertical L3
  constraint coincident L0.start L4.start
  constraint perpendicular L3 L5
  constraint perpendicular L1 L7
  constraint collinear L5 L7
  constraint coincident L0.end L1
  constraint coincident L0.start L3
  measures "d340" distance of L1.end L2.end
  measures "d341" distance of L0.end L1.end
  measures "d342" angle of L6 L7
  measures "d343" angle of L4 L5
  measures "d344" distance of L0 L7
extrude "Extrude1'''''''''" add sketch "Sketch1 (9)" along normal blind 4.7625 separate body makes body 11 in component "Pull"
sketch "Sketch2 (6)" plane through (19.05, 0, 0) normal (1, 0, 0) x (0, 0, -1) in component "Pull"
  line L0 (-17.4625, 0) -> (-7.9375, 0)
  line L1 (-7.9375, 0) -> (-7.9375, 4.7625)
  line L2 (-7.9375, 4.7625) -> (-17.4625, 4.7625)
  line L3 (-17.4625, 4.7625) -> (-17.4625, 0)
  line L4 (-17.4625, 0) -> (-7.9375, 0.7937)
  dimension "d348" = 0.7937
  constraint coincident L0.start L3.end
  constraint coincident L1 L4.end
  measures "d348" distance of L0.end L4.end
extrude "Extrude2'''''''" cut sketch "Sketch2 (6)" against normal up to surface (19.05 mm away) contours L0 L1 L4 bodies 11 in component "Pull"
draft "Draft1" angle -5 neutral plane through (19.05, 0, 17.4625) pull (0, 0, 1) 2 faces at (19.05, 1.8521, 14.2875) (0, 1.8521, 14.2875) on bodies 11 in component "Pull"
chamfer "Chamfer2" distance 1.5875 angle 45 18 edges at (254, 3.9688, 0) (127, 0, 0) (0, 3.9688, 0) (0, 0, 2.6792) (254, 0, 2.6792) (254, 0, 37.7031) (254, 0, 71.8344) (254, 0, 105.9656) (254, 0, 140.0969) (254, 0, 175.1208) (127, 0, 177.8) (254, 3.9688, 177.8) (0, 3.9688, 177.8) (0, 0, 175.1208) (0, 0, 140.0969) (0, 0, 105.9656) (0, 0, 71.8344) (0, 0, 37.7031) on bodies 3 in component "Top"
chamfer "Chamfer2'" distance 1.5875 angle 45 12 edges at (7.9375, 46.8313, 177.8) (7.9375, 93.6625, 157.1625) (7.9375, 93.6625, 123.0312) (7.9375, 93.6625, 88.9) (7.9375, 93.6625, 54.7687) (7.9375, 93.6625, 20.6375) (7.9375, 46.8312, 0) (7.9375, 0, 20.6375) (7.9375, 0, 54.7687) (7.9375, 0, 88.9) (7.9375, 0, 123.0312) (7.9375, 0, 157.1625) on bodies 2 in component "Side"
chamfer "Chamfer1'" distance 1.5875 angle 45 12 edges at (254, 7.9375, 140.0969) (254, 7.9375, 105.9656) (254, 7.9375, 71.8344) (254, 7.9375, 37.7031) (254, 11.9062, 0) (254, 11.9062, 177.8) (0, 7.9375, 37.7031) (0, 7.9375, 71.8344) (0, 7.9375, 105.9656) (0, 7.9375, 140.0969) (0, 11.9062, 177.8) (0, 11.9062, 0) on bodies 1 in component "Bottom"
chamfer "Chamfer2''" distance 1.5875 angle 45 6 edges at (0, 7.9375, 174.327) (127, 7.9375, 177.8) (127, 7.9375, 0) (0, 7.9375, 3.473) (254, 7.9375, 174.327) (254, 7.9375, 3.473) on bodies 1 in component "Bottom"
sketch "Sketch1 (10)" plane through (0, 0, 0) normal (1, 0, 0) x (0, 0, -1) in component "Wedge"
  line L0 (0, 0) -> (-7.9375, 0)
  line L1 (-7.9375, 0) -> (-7.9375, 6.35)
  line L2 (-7.9375, 6.35) -> (0, 6.35)
  line L3 (0, 6.35) -> (0, 0)
  dimension "d461" = 7.9375
  dimension "d462" = 6.35
  constraint horizontal L0
  constraint vertical L1
  constraint horizontal L2
  constraint vertical L3
  constraint coincident L0.start L3.end
  measures "d461" distance of L0.start L0.end
  measures "d462" distance of L0.end L1.end
extrude "Extrude1''''''''''" add sketch "Sketch1 (10)" along normal blind 1.5875 separate body makes body 12 in component "Wedge"
pattern_linear "00000000-0000-0000-0000-000000000000" [suppressed]
component "Bottom" placed x (1, 0, 0) y (0, 1, 0) z (0, 0, 1) at (0, 0, 0)
component "Side" placed x (1, 0, 0) y (0, 1, 0) z (0, 0, 1) at (246.0625, 7.9375, 0)
component "Top" placed x (1, 0, 0) y (0, -1, 0) z (0, 0, -1) at (0, 101.6, 177.8)
component "Divider" placed x (1, 0, 0) y (0, 1, 0) z (0, 0, 1) at (123.0312, 15.875, 7.9375)
component "Back" placed x (1, 0, 0) y (0, 1, 0) z (0, 0, 1) at (3.9688, 15.875, 0)
component "DrawerFront" placed x (1, 0, 0) y (0, 1, 0) z (0, 0, 1) at (8.7312, 15.875, 169.8625)
component "DrawerSide" placed x (1, 0, 0) y (0, 1, 0) z (0, 0, 1) at (8.7312, 15.875, 174.625)
component "DrawerBack" placed x (1, 0, 0) y (0, 1, 0) z (0, 0, 1) at (8.7312, 23.8125, 7.9375)
component "DrawerSide(Mirror)" placed x (-1, 0, 0) y (0, 1, 0) z (0, 0, -1) at (122.2375, 15.875, 174.625)
component "DrawerBottom" placed x (1, 0, 0) y (0, 1, 0) z (0, 0, 1) at (12.7, 15.875, 169.8625)
component "Pull" placed x (1, 0, 0) y (0, 1, 0) z (0, 0, 1) at (55.9594, 88.1063, 169.8625)
component "Side" placed x (-1, 0, 0) y (0, -1, 0) z (0, 0, 1) at (7.9375, 101.6, 0)
component "DrawerFront" placed x (1, 0, 0) y (0, 1, 0) z (0, 0, 1) at (131.7625, 15.875, 169.8625)
component "DrawerSide" placed x (1, 0, 0) y (0, 1, 0) z (0, 0, 1) at (131.7625, 15.875, 174.625)
component "Pull" placed x (1, 0, 0) y (0, 1, 0) z (0, 0, 1) at (178.9906, 88.1063, 169.8625)
component "DrawerBottom" placed x (1, 0, 0) y (0, 1, 0) z (0, 0, 1) at (135.7313, 15.875, 169.8625)
component "DrawerBack" placed x (1, 0, 0) y (0, 1, 0) z (0, 0, 1) at (131.7625, 23.8125, 7.9375)
component "DrawerSide(Mirror)" placed x (-1, 0, 0) y (0, 1, 0) z (0, 0, -1) at (245.2688, 15.875, 174.625)
component "Wedge" placed x (1, 0, 0) y (0, 1, 0) z (0, 0, 1) at (124.2219, 95.25, 25.6646)
component "Wedge" placed x (1, 0, 0) y (0, 1, 0) z (0, 0, 1) at (124.2219, 95.25, 84.9312)
component "Wedge" placed x (1, 0, 0) y (0, 1, 0) z (0, 0, 1) at (124.2219, 95.25, 144.1979)
component "Wedge" placed x (1, 0, 0) y (0, 1, 0) z (0, 0, 1) at (124.2219, 7.9375, 25.6646)
component "Wedge" placed x (-1, 0, 0) y (0, -1, 0) z (0, 0, 1) at (125.8094, 14.2875, 84.9312)
component "Wedge" placed x (-1, 0, 0) y (0, -1, 0) z (0, 0, 1) at (125.8094, 14.2875, 144.1979)
component "Wedge" placed x (1, 0, 0) y (0, 1, 0) z (0, 0, 1) at (128.1906, 95.25, 25.6646)
component "Wedge" placed x (1, 0, 0) y (0, 1, 0) z (0, 0, 1) at (128.1906, 95.25, 84.9312)
component "Wedge" placed x (1, 0, 0) y (0, 1, 0) z (0, 0, 1) at (128.1906, 95.25, 144.1979)
component "Wedge" placed x (-1, 0, 0) y (0, -1, 0) z (0, 0, 1) at (129.7781, 14.2875, 25.6646)
component "Wedge" placed x (-1, 0, 0) y (0, -1, 0) z (0, 0, 1) at (129.7781, 14.2875, 84.9312)
component "Wedge" placed x (-1, 0, 0) y (0, -1, 0) z (0, 0, 1) at (129.7781, 14.2875, 144.1979)
equation "thickness = ( 5 / 16 ) * 1 in"
equation "width = 10 in"
equation "depth = 7 in"
equation "height = 4 in"
equation "bottom_thickness = ( 5 / 8 ) * 1 in"
equation "drawer_reveal = ( 1 / 32 ) * 1 in"
equation "dovetail_angle = 18 deg"
equation "d8 = width"
equation "d9 = depth"
equation "d10 = bottom_thickness"
equation "d12 = 90 deg - dovetail_angle"
equation "d13 = d12"
equation "dovetail_count = 5"
equation "d15 = dovetail_count"
equation "d17 = ( depth - dovetail_width ) / 2 - pin_width"
equation "dovetail_width = 1 in"
equation "pin_width = ( 5 / 16 ) * 1 in"
equation "d22 = dovetail_width"
equation "d23 = thickness"
equation "d24 = -thickness"
equation "d27 = thickness"
equation "d30 = depth / 3"
equation "divider_tenonCount = 3"
equation "d35 = height - bottom_thickness + thickness"
equation "d36 = thickness"
equation "d37 = depth"
equation "d40 = dovetail_count"
equation "d42 = ( depth - dovetail_width ) / 2 - pin_width"
equation "d44 = 90 deg - dovetail_angle"
equation "d45 = d12"
equation "d46 = dovetail_width"
equation "d47 = thickness"
equation "d8_1 = width"
equation "d9_1 = depth"
equation "d10_1 = thickness"
equation "d12_1 = 90 deg - dovetail_angle"
equation "d13_1 = d12_1"
equation "d15_1 = dovetail_count"
equation "d17_1 = ( depth - dovetail_width ) / 2 - pin_width"
equation "d22_1 = dovetail_width"
equation "d23_1 = thickness"
equation "d24_1 = -thickness"
equation "d27_1 = thickness"
equation "d30_1 = depth / 3"
equation "d87 = depth - thickness"
equation "d88 = height - bottom_thickness - thickness"
equation "d89 = thickness"
equation "d90 = depth / 2"
equation "d92 = divider_tenonCount"
equation "d94 = depth / 3"
equation "d96 = thickness"
equation "d99 = thickness"
equation "d100 = divider_tenonCount"
equation "d102 = depth / 3"
equation "wedge_thickness = ( 1 / 16 ) * 1 in"
equation "d105 = wedge_thickness"
equation "d106 = 0.8 * thickness"
equation "d107 = wedge_thickness"
equation "d108 = thickness * 0.8"
equation "d123 = -thickness"
equation "d149 = width - thickness"
equation "d150 = height - thickness - bottom_thickness"
equation "d151 = thickness"
equation "foot_width = 1 in"
equation "d166 = foot_width"
equation "d167 = -foot_height"
equation "foot_height = bottom_thickness - thickness"
equation "d171 = foot_height / 2"
equation "d172 = bead_flat"
equation "bead_flat = ( 1 / 32 ) * 1 in"
equation "blindDovetail_depth = thickness - ( 1 / 8 ) * 1 in"
equation "d187 = drawer_height"
equation "d188 = drawer_width"
equation "d189 = thickness"
equation "d191 = blindDovetail_depth"
equation "d192 = 90 deg + dovetail_angle"
equation "d193 = d192"
equation "drawer_frontDovetailWidth = ( 11 / 16 ) * 1 in"
equation "drawer_frontPinWidth = 0.25 in"
equation "drawer_dovetailCount = 3"
equation "d197 = drawer_frontDovetailWidth"
equation "drawer_height = height - thickness - bottom_thickness - drawer_reveal"
equation "drawer_width = ( width - 3 * thickness ) / 2 - 2 * drawer_reveal"
equation "d202 = ( drawer_height - drawer_frontDovetailWidth ) / 2 - drawer_frontPinWidth"
equation "d204 = -thickness"
equation "pull_width = 0.75 in"
equation "d208 = pull_width"
equation "d209 = 90 deg + dovetail_angle"
equation "d210 = d209"
equation "d211 = -pull_thickness"
equation "pull_thickness = ( 3 / 16 ) * 1 in"
equation "pull_length = ( 3 / 8 ) * 1 in"
equation "d215 = drawer_reveal"
equation "d216 = drawer_height"
equation "d217 = depth - 2 * thickness + blindDovetail_depth"
equation "d218 = thickness"
equation "d222 = ( drawer_height - drawer_frontDovetailWidth ) / 2 - drawer_frontPinWidth"
equation "d224 = blindDovetail_depth"
equation "d225 = 90 deg + dovetail_angle"
equation "d226 = d192"
equation "d227 = drawer_frontDovetailWidth"
equation "d230 = ( drawer_height - drawer_backDovetailWidth ) / 2 - drawer_backPinWidth"
equation "d232 = thickness"
equation "d233 = 90 deg + dovetail_angle"
equation "d234 = d192"
equation "d235 = drawer_backDovetailWidth"
equation "drawer_backDovetailWidth = ( 9 / 16 ) * 1 in"
equation "drawer_backPinWidth = thickness"